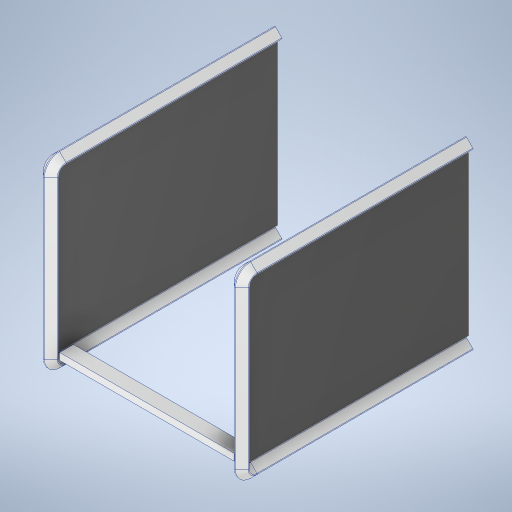
# Autodesk Inventor part: Frame Test
Saved by Autodesk Inventor 2024 (Build 280153000, 153)
## iProperties
Created: 2024-11-19
Part Number: Frame Test
Material: Aluminum 6061
Document SubType Name: Modeling
Designer: Ishaan
Density: 2.7 g/cm^3
Appearance: Aluminum - Flat
Author: Ishaan
Autodesk Inventor part; units mm, degrees
ref_plane "YZ Plane" through (0, 0, 0) normal (1, 0, 0) x (0, 1, 0)
ref_plane "XZ Plane" through (0, 0, 0) normal (0, 1, 0) x (-1, 0, 0)
sketch "Sketch1" plane through (0, 0, 0) normal (0, 0, 1) x (1, 0, 0)
  line L0 (276.5, -251.5) -> (-276.5, -251.5) construction
  line L1 (-276.5, -251.5) -> (-276.5, 251.5) construction
  line L2 (-276.5, 251.5) -> (276.5, 251.5) construction
  line L3 (276.5, 251.5) -> (276.5, -251.5) construction
  line L4 (276.5, -251.5) -> (-276.5, 251.5) construction
  line L5 (-276.5, -251.5) -> (276.5, 251.5) construction
  line L6 (275.0858, 231.701) -> (256.701, 250.0858)
  line L7 (256.701, 252.9142) -> (275.0858, 271.299)
  line L8 (277.9142, 271.299) -> (296.299, 252.9142)
  line L9 (296.299, 250.0858) -> (277.9142, 231.701)
  line L10 (276.5, 230.2868) -> (276.5, 272.7132) construction
  line L11 (255.2868, 251.5) -> (297.7132, 251.5) construction
  arc A0 (256.701, 252.9142) -> (256.701, 250.0858) centre (258.1152, 251.5) ccw
  arc A1 (277.9142, 271.299) -> (275.0858, 271.299) centre (276.5, 269.8848) ccw
  arc A2 (296.299, 250.0858) -> (296.299, 252.9142) centre (294.8848, 251.5) ccw
  arc A3 (275.0858, 231.701) -> (277.9142, 231.701) centre (276.5, 233.1152) ccw
  point P0 (0, 0)
  dimension "d0" = 553
  dimension "d1" = 503
  dimension "d2" = 30
  dimension "d3" = 2
  constraints: 24 end point, 8 point on circle, 8 point on line, 8 tangent, 4 centre point, 4 midpoint, 4 parallel, 3 equal radius, 2 collinear, 2 perpendicular, 1 horizontal
  measures "d0" distance of L1.end L2.end
  measures "d1" distance of L0.end L1.end
  measures "d2" distance of L10.end L11.end
  measures "d3" radius of A0
extrude "Extrusion1" add sketch "Sketch1" along normal blind 625
mirror "Mirror1" about plane through (0, 0, 0) normal (1, 0, 0) of "Extrusion1"
mirror "Mirror2" about plane through (0, 0, 0) normal (0, 1, 0) of "Extrusion1", "Mirror1"
ref_plane "Work Plane1" through (-276.5, -251.5, 0) normal (1, 0, 0) x (0, 1, 0)
sketch "Sketch2" plane through (-276.5, -251.5, 0) normal (1, 0, 0) x (0, 1, 0)
  line L0 (523.3848, 625) -> (523.3848, 0) projected
  line L1 (523.3848, 0) -> (482.6152, 0) projected
  line L2 (482.6152, 0) -> (482.6152, 625) projected
  line L3 (482.6152, 625) -> (523.3848, 625) projected
  line L4 (-20.3848, 0) -> (-20.3848, 625) projected
  line L5 (-20.3848, 625) -> (20.3848, 625) projected
  line L6 (20.3848, 625) -> (20.3848, 0) projected
  line L7 (20.3848, 0) -> (-20.3848, 0) projected
  line L8 (479, 649) -> (24, 649)
  arc A0 (503, 625) -> (479, 649) centre (479, 625) ccw
  arc A1 (24, 649) -> (0, 625) centre (24, 625) ccw
  line L9 (24, 628.6152) -> (479, 628.6152) construction
  line L10 (479, 628.6152) -> (479, 669.3848) construction
  line L11 (479, 669.3848) -> (24, 669.3848) construction
  line L12 (24, 669.3848) -> (24, 628.6152) construction
  line L13 (24, 628.6152) -> (479, 669.3848) construction
  line L14 (479, 628.6152) -> (24, 669.3848) construction
  line L15 (21.5, 607.5) -> (41.5, 607.5)
  line L16 (41.5, 607.5) -> (41.5, 647.5)
  line L17 (41.5, 647.5) -> (21.5, 647.5)
  line L18 (21.5, 647.5) -> (21.5, 607.5)
  line L19 (41.5, 607.5) -> (1.5, 607.5)
  line L20 (1.5, 607.5) -> (1.5, 627.5)
  line L21 (1.5, 627.5) -> (41.5, 627.5)
  line L22 (41.5, 627.5) -> (41.5, 607.5)
  point P0 (251.5, 0)
  point P1 (251.5, 649)
  dimension "d8" = 455
  dimension "d16" = 20
  dimension "d17" = 40
  dimension "d18" = 40
  dimension "d19" = 20
  dimension "d20" = 1.5
  dimension "d21" = 1.5
  dimension "d22" = 2.5
  constraints: 30 end point, 6 parallel, 5 midpoint, 4 horizontal, 4 perpendicular, 4 point on circle, 2 centre point, 2 line through centre, 2 tangent, 1 point on line
  measures "d8" distance of L8.start L8.end
  measures "d16" distance of L17.end L16.end
  measures "d17" distance of L16.end L15.end
  measures "d18" distance of L20.end L21.end
  measures "d19" distance of L19.end L20.end
  measures "d20" distance between parallel lines of L8 L17
  measures "d21" distance from line of A1.end L20
  measures "d22" distance between parallel lines of L21 L5
sketch "Sketch3" plane through (-276.5, -269.8848, 625) normal (0, 0, 1) x (1, 0, 0)
  line L0 (-19.799, 16.9706) -> (-1.4142, -1.4142) projected
  arc A0 (-1.4142, -1.4142) -> (1.4142, -1.4142) centre (0, 0) ccw projected
  line L1 (1.4142, -1.4142) -> (19.799, 16.9706) projected
  arc A1 (19.799, 16.9706) -> (19.799, 19.799) centre (18.3848, 18.3848) ccw projected
  line L2 (19.799, 19.799) -> (1.4142, 38.1838) projected
  arc A2 (1.4142, 38.1838) -> (-1.4142, 38.1838) centre (0, 36.7696) ccw projected
  line L3 (-1.4142, 38.1838) -> (-19.799, 19.799) projected
  arc A3 (-19.799, 19.799) -> (-19.799, 16.9706) centre (-18.3848, 18.3848) ccw projected
  point P0 (276.5, 269.8848)
sweep "Sweep1" add profiles "Sketch3" path "Sketch2" path curves A1 L8 A0
mirror "Mirror3" about plane through (0, 0, 0) normal (1, 0, 0) of "Sweep1"
sketch "Sketch4" plane through (-276.5, -251.5, 0) normal (1, 0, 0) x (0, 1, 0)
  arc A0 (523.3848, 625) -> (479, 669.3848) centre (479, 625) ccw projected
  line L0 (523.3848, 625) -> (523.3848, 0) projected
  line L1 (523.3848, 0) -> (482.6152, 0) projected
  line L2 (482.6152, 0) -> (482.6152, 625) projected
  arc A1 (482.6152, 625) -> (479, 628.6152) centre (479, 625) ccw projected
  line L3 (479, 628.6152) -> (24, 628.6152) projected
  arc A2 (24, 628.6152) -> (20.3848, 625) centre (24, 625) ccw projected
  line L4 (20.3848, 625) -> (20.3848, 0) projected
  line L5 (20.3848, 0) -> (-20.3848, 0) projected
  line L6 (-20.3848, 0) -> (-20.3848, 625) projected
  arc A3 (24, 669.3848) -> (-20.3848, 625) centre (24, 625) ccw projected
  line L7 (24, 669.3848) -> (479, 669.3848) projected
  arc A4 (24, 627.5) -> (21.5, 625) centre (24, 625) ccw
  line L8 (24, 627.5) -> (479, 627.5)
  arc A5 (481.5, 625) -> (479, 627.5) centre (479, 625) ccw
  line L9 (481.5, 625) -> (481.5, -1.1152)
  line L10 (481.5, -1.1152) -> (524.5, -1.1152)
  line L11 (524.5, -1.1152) -> (524.5, 625)
  arc A6 (524.5, 625) -> (479, 670.5) centre (479, 625) ccw
  line L12 (479, 670.5) -> (24, 670.5)
  arc A7 (24, 670.5) -> (-21.5, 625) centre (24, 625) ccw
  line L13 (-21.5, 625) -> (-21.5, -1.1152)
  line L14 (-21.5, -1.1152) -> (21.5, -1.1152)
  line L15 (21.5, -1.1152) -> (21.5, 625)
  line L16 (481.5, -1.1152) -> (21.5, -1.1152)
  line L17 (21.5, -1.1152) -> (21.5, -6.35)
  line L18 (21.5, -6.35) -> (481.5, -6.35)
  line L19 (481.5, -6.35) -> (481.5, -1.1152)
  point P0 (251.5, 0)
  dimension "d11" = 460
  dimension "d12" = 1.1152
  dimension "d13" = 6.35
  constraints: 24 end point, 8 point on circle, 4 centre point, 2 parallel, 1 collinear, 1 horizontal, 1 perpendicular, 11 other
  measures "d11" distance between parallel lines of L15 L9
  measures "d12" distance between parallel lines of L15 L4
  measures "d13" distance between parallel lines of L18 L5
extrude "Extrusion2" add sketch "Sketch4" along normal mid plane 3 separate body contours L8 A5 L9 L16 L15 A4 | L16 L19 L18 L17
mirror "Mirror4" about plane through (0, 0, 0) normal (1, 0, 0) of "Extrusion2" bodies 2
sketch "Sketch5" plane through (0, 0, 0) normal (1, 0, 0) x (0, 1, 0)
  line L0 (-210, 607.5) -> (-210, 647.5) projected
  line L1 (-210, 607.5) -> (-250, 607.5) projected
  line L2 (-210, 607.5) -> (-230, 607.5)
  line L3 (-230, 607.5) -> (-230, 647.5)
  line L4 (-230, 647.5) -> (-210, 647.5)
  line L5 (-210, 647.5) -> (-210, 607.5)
  line L6 (-210, 607.5) -> (-250, 607.5)
  line L7 (-250, 607.5) -> (-250, 627.5)
  line L8 (-250, 627.5) -> (-210, 627.5)
  line L9 (-210, 627.5) -> (-210, 607.5)
  point P0 (0, 0)
  point P1 (-230, 627.5)
  point P2 (-250, 607.5)
  dimension "d23" = 20
  dimension "d24" = 40
  dimension "d25" = 40
  dimension "d26" = 20
  constraints: 16 end point, 4 parallel, 2 horizontal, 2 perpendicular
  measures "d23" distance of L3.end L4.end
  measures "d24" distance of L2.end L3.end
  measures "d25" distance of L7.end L8.end
  measures "d26" distance of L6.end L7.end
extrude "Extrusion3" add sketch "Sketch5" along normal mid plane 505 separate body
body "Solid1"
body "Solid3"
